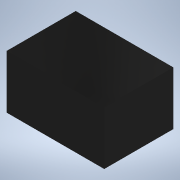
# Autodesk Inventor part: tenergy_nimh_2200
Saved by Autodesk Inventor 2020.3 (Build 243373000, 373)
## iProperties
Created: 2020-11-24
Part Number: tenergy_nimh_2200
Material: Acetal Resin, Black
Document SubType Name: Modeling
Designer: Devin
Density: 1.425 g/cm^3
Appearance: Smooth - Black
Mass: 255 g
Surface Area: 156.115 cm^2
Volume: 119.934 cm^3
Author: Devin
Autodesk Inventor part; units mm, degrees
ref_plane "YZ Plane" through (0, 0, 0) normal (1, 0, 0) x (0, 1, 0)
ref_plane "XZ Plane" through (0, 0, 0) normal (0, 1, 0) x (-1, 0, 0)
ref_plane "XY Plane" through (0, 0, 0) normal (0, 0, 1) x (1, 0, 0)
sketch "Sketch1" plane through (0, 0, 0) normal (0, 1, 0) x (-1, 0, 0)
  line L0 (0, 0) -> (-72.3, 0)
  line L1 (-72.3, 0) -> (-72.3, -51.2)
  line L2 (-72.3, -51.2) -> (0, -51.2)
  line L3 (0, -51.2) -> (0, 0)
  dimension "d0" = 72.3
  dimension "d1" = 51.2
  constraints: 8 end point, 2 parallel, 1 horizontal, 1 perpendicular
  measures "d0" distance of L0.start L0.end
  measures "d1" distance of L1.end L0.end
extrude "Extrusion1" add sketch "Sketch1" along normal blind 29.5
body "Solid1"
